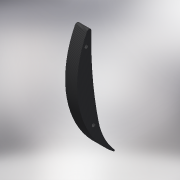
# Autodesk Inventor part: styro_50_main
Saved by Autodesk Inventor 2018.2 (Build 222227000, 227)
## iProperties
Created: 2017-12-11
Part Number: styro_50_main
Material: ポリスチレン、耐衝撃性
Document SubType Name: Modeling
Designer: kuwano
Density: 1.022 g/cm^3
Appearance: カーボンファイバー
Mass: 1214.74 g
Surface Area: 1128.2 cm^2
Volume: 1188.59 cm^3
Author: kuwano
Autodesk Inventor part; units mm, degrees
ref_plane "YZ Plane" through (0, 0, 0) normal (1, 0, 0) x (0, 1, 0)
ref_plane "XZ Plane" through (0, 0, 0) normal (0, 1, 0) x (-1, 0, 0)
ref_plane "XY Plane" through (0, 0, 0) normal (0, 0, 1) x (1, 0, 0)
sketch "スケッチ1" plane through (0, 0, 0) normal (1, 0, 0) x (0, 1, 0)
  line L0 (-8.1429, 150) -> (114.6125, -400)
  line L1 (-14.3507, 287.6765) -> (28.2901, -658.0026)
  arc A0 (-8.1429, 150) -> (21.0831, -240) centre (1567.8058, 72.0039) ccw
  arc A1 (21.0831, -240) -> (114.6125, -400) centre (301.453, -183.444) ccw
  arc A2 (-8.1429, 150) -> (-17.4923, 133.9393) centre (678.5198, -260.4806) ccw
  arc A3 (-17.4923, 133.9393) -> (114.6125, -400) centre (330.5138, -63.2706) ccw
  point P0 (0, 0)
  point P1 (-8.1429, -100)
  point P2 (-14.3507, 287.6765)
  point P3 (28.2901, -658.0026)
  dimension "d0" = 10
  dimension "d1" = 550
  dimension "d2" = 250
  dimension "d3" = 1577.8776
  dimension "d4" = 286.0172
  dimension "d5" = 160
  dimension "d6" = 800
  dimension "d21" = 400
  constraints: 8 point on circle, 4 centre point, 2 end point, 2 tangent, 4 other
  measures "d1" vertical distance of L0.end L0.start
  measures "d2" distance of point (-8.143, -100) L0.start
  measures "d3" radius of A0
  measures "d4" radius of A1
  measures "d5" vertical distance of L0.end A0.end
  measures "d6" radius of A2
  measures "d21" radius of A3
extrude "押し出し1" add sketch "スケッチ1" along normal mid plane 50 contours A0 L1 A3 A2 | A3 L1 A0 A1
fillet "フィレット1" radius 10 1 edges at (0, -8.1429, 150)
fillet "フィレット1" radius 3 1 edges at (0, 114.6125, -400)
sketch "スケッチ2" plane through (25, 0, 0) normal (1, 0, 0) x (0, 0, -1)
  circle A0 centre (-60, -30) radius 7.5
  circle A1 centre (240, 0) radius 7.5
  point P0 (0, 0)
  dimension "d11" = 15
  dimension "d12" = 15
  dimension "d13" = 300
  dimension "d16" = 30
  dimension "d19" = 30
  dimension "d20" = 60
  constraints: 2 centre point
  measures "d11" diameter of A1
  measures "d12" diameter of A0
  measures "d13" horizontal distance of A1.centre A0.centre
  measures "d16" vertical distance of A1.centre A0.centre
  measures "d19" vertical distance of A0.centre point (0, 0)
  measures "d20" horizontal distance of A0.centre point (0, 0)
extrude "押し出し2" cut sketch "スケッチ2" against normal through all
